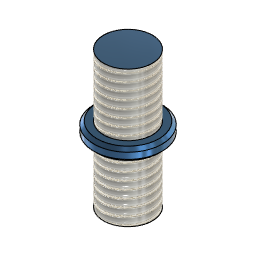
stp2_v39 (Autodesk Fusion 360 archive; units mm, degrees)
design "screw 3"
Autodesk Fusion 360 part; units mm, degrees
sketch "Sketch1" plane through (0, 0, 0) normal (0, 0, 1) x (1, 0, 0)
  circle A0 centre (0, 0) radius 4
  circle A1 centre (0, 0) radius 5.5
  dimension "d1" = 8
  dimension "d2" = 1.5
  constraint coincident A0.centre A1.centre
  measures "d1" diameter of A0
extrude "Extrude1" add sketch "Sketch1" along normal mid plane 2 contours A0 | A1
extrude "Extrude2" add sketch "Sketch1" along normal mid plane 22 contours A0
thread "Thread1" "ISO Metric profile 8.0 M8x1.25 6g" major diameter 7.866 minor diameter 6.4455 pitch 1.25 angle 60 resizes the face on face at (3.9801, -0.3983, -4.3333)
thread "Thread2" "ISO Metric profile 8.0 M8x1.25 6g" major diameter 7.866 minor diameter 6.4455 pitch 1.25 angle 60 resizes the face on face at (3.995, 0.1994, 4.3333)
chamfer "Chamfer1" distance 0.5 angle 45 2 edges at (-5.1278, -1.9889, 1) (-5.1278, 1.9889, -1)

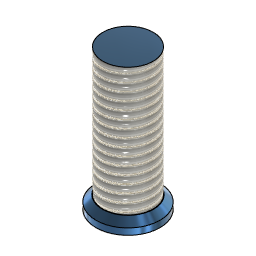
design "screw2"
Autodesk Fusion 360 part; units mm, degrees
sketch "Sketch1" plane through (0, 0, 0) normal (0, 0, 1) x (1, 0, 0)
  circle A0 centre (0, 0) radius 4
  circle A1 centre (0, 0) radius 5
  dimension "d1" = 8
  dimension "d2" = 1
  constraint coincident A0.centre A1.centre
  measures "d1" diameter of A0
extrude "Extrude1" add sketch "Sketch1" along normal blind 20 contours A0
thread "Thread1" "ISO Metric profile 8.0 M8x1.25 6g" major diameter 7.866 minor diameter 6.4455 pitch 1.25 angle 60 resizes the face on face at (3.995, -0.1994, 13.3333)
extrude "Extrude3" add sketch "Sketch1" against normal blind 2 contours A0 | A1
chamfer "Chamfer1" distance 1 angle 45 1 edges at (-4.6616, -1.8081, 0)
sketch "Sketch2" plane through (0, 0, -2) normal (0, 0, -1) x (1, 0, 0)
  circle A0 centre (0, 0) radius 5
  line L0 (-0.5, 4) -> (0.5, 4)
  line L1 (0.5, -4) -> (-0.5, -4)
  line L2 (4, 0.5) -> (4, -0.5)
  line L3 (-4, -0.5) -> (-4, 0.5)
  line L4 (-0.5, -4) -> (-0.5, -0.5)
  line L5 (-0.5, 0.5) -> (-0.5, 4)
  line L6 (-4, 0.5) -> (-0.5, 0.5)
  line L7 (0.5, 0.5) -> (4, 0.5)
  line L8 (0.5, 4) -> (0.5, 0.5)
  line L9 (0.5, -0.5) -> (0.5, -4)
  line L10 (4, -0.5) -> (0.5, -0.5)
  line L11 (-0.5, -0.5) -> (-4, -0.5)
  constraint horizontal L0
  constraint vertical L8
  constraint horizontal L1
  constraint vertical L4
  constraint horizontal L6
  constraint vertical L2
  constraint horizontal L10
  constraint vertical L3
  constraint coincident L4.end L10
  constraint collinear L4 L5
  constraint collinear L6 L7
  constraint collinear L8 L9
  constraint collinear L10 L11
extrude "Extrude4" cut sketch "Sketch2" against normal blind 0.5 contours L0 L1 L2 L3 L4 L5 L6 L7 L8 L9 L10 L11

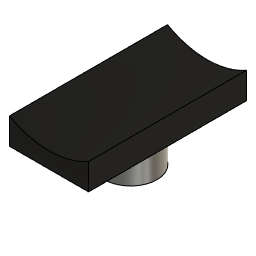
design "holder"
Autodesk Fusion 360 part; units mm, degrees
sketch "Sketch1" plane through (0, 0, 0) normal (0, 0, 1) x (1, 0, 0)
  circle A0 centre (0, 0) radius 4
  circle A1 centre (0, 0) radius 5
  dimension "d1" = 8
  dimension "d2" = 1
  constraint coincident A0.centre A1.centre
  measures "d1" diameter of A0
extrude "Extrude1" add sketch "Sketch1" along normal blind 6.5 makes body 1
thread "Thread1" "ISO Metric profile 8.0 M8x1.25 6H" major diameter 8.17 minor diameter 6.7795 pitch 1.25 angle 60 resizes the face on face at (3.9801, -0.3983, 4.3333) on bodies 1
sketch "Sketch2" plane through (0, 0, 6.5) normal (0, 0, 1) x (-1, 0, 0)
  circle A0 centre (0, 0) radius 3.3898
  circle A1 centre (0, 0) radius 5
  line L0 (-14.5, 5) -> (14.5, 5)
  line L1 (14.5, 5) -> (14.5, -5)
  line L2 (14.5, -5) -> (-14.5, -5)
  line L3 (-14.5, -5) -> (-14.5, 5)
  line L4 (-14.5, 5) -> (14.5, -5) construction
  line L5 (14.5, 5) -> (-14.5, -5) construction
  constraint horizontal L0
  constraint perpendicular L0 L1
  constraint parallel L0 L2
  constraint parallel L1 L3
  constraint coincident L4 A0.centre
  constraint coincident L5 A0.centre
  constraint coincident A0.centre A1.centre
hole "Hole1" at (0, 0, 0) direction (0, 0, 1) diameter 6.78 depth 6.5 tip angle 118 bodies 1
thread "Thread2" "ISO Metric profile 8.0 M8x1.25 6H"
sketch "Sketch5" plane through (0, 0, 6.5) normal (0, 0, 1) x (-1, 0, 0)
  circle A0 centre (0, 0) radius 3.3898
  circle A1 centre (0, 0) radius 5
  circle A2 centre (0, -4.2) radius 0.3
  circle A3 centre (3.6373, -2.1) radius 0.3
  circle A4 centre (3.6373, 2.1) radius 0.3
  circle A5 centre (0, 4.2) radius 0.3
  circle A6 centre (-3.6373, 2.1) radius 0.3
  circle A7 centre (-3.6373, -2.1) radius 0.3
  dimension "d27" = 360
extrude "Extrude7" cut sketch "Sketch5" against normal blind 2 draft -5 contours A2 | A3 | A4 | A5 | A6 | A7 bodies 1
sketch "Sketch6" plane through (0, 0, 0) normal (0, 0, 1) x (1, 0, 0)
  line L0 (35, 15) -> (15, 15)
  line L1 (15, 15) -> (15, -15)
  line L2 (15, -15) -> (35, -15)
  line L3 (35, -15) -> (35, 15)
  line L4 (35, 15) -> (15, -15) construction
  line L5 (15, 15) -> (35, -15) construction
  point P0 (25, 0)
  dimension "d30" = 20
  dimension "d31" = 30
  constraint horizontal L0
  constraint perpendicular L0 L1
  constraint parallel L0 L2
  constraint parallel L1 L3
  constraint coincident L4 P0
  constraint coincident L5 P0
  measures "d30" distance of L1.end L2.end
  measures "d31" distance of L0.end L1.end
extrude "Extrude8" add sketch "Sketch6" along normal blind 5 separate body makes body 2
move_face "OffsetFaces1" offset -5 1 faces at (35, -5, 1.6667) on bodies 2
sketch "Sketch7" plane through (0, -15, 0) normal (0, -1, 0) x (1, 0, 0)
  line L0 (15, 0) -> (30, 0)
  line L1 (30, 0) -> (30, 5)
  line L2 (30, 5) -> (15, 5)
  line L3 (15, 5) -> (15, 0)
  line L4 (22.5, 5) -> (22.5, 21)
  line L5 (15, 5) -> (22.5, 17.9904)
  line L6 (30, 5) -> (22.5, 17.9904)
  spline S0 degree 5 poles (15, 5) (15.109, 5.0688) (15.3315, 5.201) (15.6789, 5.3824) (16.1695, 5.5908) (16.8286, 5.7953) (17.5334, 5.9451) (18.2823, 6.044) (19.0719, 6.0995) (19.8963, 6.123) (20.7483, 6.127) (21.6193, 6.1234) (22.5, 6.1209) (23.3807, 6.1234) (24.2517, 6.127) (25.1037, 6.123) (25.9281, 6.0995) (26.7177, 6.044) (27.4666, 5.9451) (28.1714, 5.7953) (28.8305, 5.5908) (29.3211, 5.3824) (29.6685, 5.201) (29.891, 5.0688) (30, 5) knots 0 0 0 0 0 0 0.05 0.1 0.15 0.2 0.25 0.3 0.35 0.4 0.45 0.5 0.55 0.6 0.65 0.7 0.75 0.8 0.85 0.9 0.95 1 1 1 1 1 1
  point P0 (18, 6)
  point P1 (22.5, 6.1221)
  point P2 (27, 6)
  dimension "d35" = 15
  constraint midpoint L2 L4.start
  constraint perpendicular L2 L4
  constraint coincident L2.end L3.start
  constraint coincident L4 L5.end
  constraint coincident L1.end L2.start
  constraint coincident L4 P1
  measures "d35" distance of L2.end L5.end
extrude "Extrude9" cut sketch "Sketch7" against normal blind 33.5 contours L2 L4 S0 | L2 L4 S0 bodies 2
move_body "Move1" bodies 2 to x (1, 0, 0) y (0, 1, 0) z (0, 0, 1) at (-23, 0, 16)
sketch "Sketch8" plane through (0, 0, 16) normal (0, 0, -1) x (1, 0, 0)
  line L0 (7, -15) -> (7, 15)
  line L1 (7, 15) -> (-8, 15)
  line L2 (-8, 15) -> (-8, -15)
  line L3 (-8, -15) -> (7, -15)
  circle A0 centre (0, 0) radius 3.5
  circle A1 centre (0, 0) radius 5
  circle A2 centre (0, 4.2) radius 0.3
  circle A3 centre (-3.6373, 2.1) radius 0.3
  circle A4 centre (-3.6373, -2.1) radius 0.3
  circle A5 centre (0, -4.2) radius 0.3
  circle A6 centre (3.6373, -2.1) radius 0.3
  circle A7 centre (3.6373, 2.1) radius 0.3
  dimension "d39" = 360
  constraint coincident A0.centre A1.centre
  constraint concentric A0 A1
extrude "Extrude10" add sketch "Sketch8" along normal blind 2 draft -5 contours A2 | A3 | A4 | A5 | A6 | A7 bodies 2
copy_body "Body->Comp1" bodies 2 removing the originals makes body 3 in component "Component"
move_body "Move1'" bodies 3 to x (1, 0, 0) y (0, 1, 0) z (0, 0, 1) at (-13, 0, 0) in component "Component"
sketch "Sketch9" plane through (0, -15, 0) normal (0, -1, 0) x (1, 0, 0)
  line L0 (-8, 6.5) -> (7, 6.5)
  line L1 (7, 6.5) -> (7, 11.5)
  line L2 (7, 11.5) -> (-8, 11.5)
  line L3 (-8, 11.5) -> (-8, 6.5)
  arc A0 (-8, 11.5) -> (7, 11.5) centre (-0.5, 24.6157) ccw
extrude "Extrude1'" cut sketch "Sketch9" against normal blind 35 contours L2 A0 sketch seen with x (1, 0, 0) y (0, 1, 0) z (0, 0, 1) at (-13, 0, 9.5) bodies 3 in component "Component"
component "Component" placed x (1, 0, 0) y (0, 1, 0) z (0, 0, 1) at (13, 0, -9.5)
